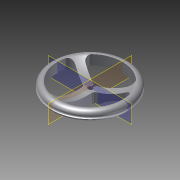
# Autodesk Inventor part: Rueda1
Saved by Autodesk Inventor 2012 (Build 160160000, 160)
## iProperties
Created: 2012-12-03
Part Number: Rueda1
Material: Default
Document SubType Name: Modeling
Designer: ALUMNO
Density: 1 g/cm^3
Author: ALUMNO
Autodesk Inventor part; units mm, degrees
ref_plane "XY Plane" through (0, 0, 0) normal (0, 0, 1) x (1, 0, 0)
sketch "Sketch1" plane through (0, 0, 0) normal (0, 0, 1) x (1, 0, 0)
  line L0 (-20, 0) -> (20, 0) construction
  line L1 (-1.118, -1) -> (1.118, -1)
  line L2 (0, -3.5) -> (0, -10.5) construction
  line L3 (0, 42) -> (0, -42) construction
  line L4 (3, -1.8028) -> (3, -19.7737)
  line L5 (-3, -1.8028) -> (-3, -19.7737)
  line L6 (3.0311, 1.75) -> (9.0933, 5.25) construction
  line L7 (-3.0311, 1.75) -> (-9.0933, 5.25) construction
  line L8 (3.4347, -0.6728) -> (18.3556, 7.9418)
  line L9 (1.1347, 3.3109) -> (16.0556, 11.9255)
  arc A0 (3, -19.7737) -> (18.3556, 7.9418) centre (0, 0) ccw
  line L10 (-16.0556, 11.9255) -> (-1.1347, 3.3109)
  line L11 (-18.3556, 7.9418) -> (-3.4347, -0.6728)
  arc A1 (16.0556, 11.9255) -> (-16.0556, 11.9255) centre (0, 0) ccw
  arc A2 (-18.3556, 7.9418) -> (-3, -19.7737) centre (0, 0) ccw
  arc A3 (-3.4347, -0.6728) -> (-3, -1.8028) centre (0, 0) ccw
  arc A4 (3, -1.8028) -> (3.4347, -0.6728) centre (0, 0) ccw
  line L12 (0, 0) -> (2.0417, 7.6198) construction
  line L13 (0, 0) -> (-1.8775, 7.0067) construction
  line L14 (0.3882, 1.4489) -> (0.9059, 3.3807)
  line L15 (-0.3882, 1.4489) -> (-0.9059, 3.3807)
  arc A5 (1.1347, 3.3109) -> (0.9059, 3.3807) centre (0, 0) ccw
  arc A6 (-0.9059, 3.3807) -> (-1.1347, 3.3109) centre (0, 0) ccw
  arc A7 (1.118, -1) -> (0.3882, 1.4489) centre (0, 0) ccw
  arc A8 (-0.3882, 1.4489) -> (-1.118, -1) centre (0, 0) ccw
  circle A9 centre (0, 0) radius 30
  dimension "d3" = 1
  dimension "d4" = 3
  dimension "d5" = 3
  dimension "d8" = 360
  dimension "d10" = 2.3
  dimension "d11" = 2.3
  dimension "d12" = 2.3
  dimension "d13" = 2.3
  dimension "d14" = 20
  dimension "d15" = 20
  dimension "d16" = 20
  dimension "d17" = 3.5
  dimension "d18" = 3.5
  dimension "d19" = 15
  dimension "d20" = 15
  dimension "d21" = 3.5
  dimension "d22" = 3.5
  dimension "d23" = 1.5
  dimension "d24" = 1.5
  dimension "d25" = 60
  constraints: 30 end point, 21 point on circle, 10 centre point, 7 parallel, 5 point on line, 4 coincident, 1 collinear, 1 horizontal, 1 midpoint, 1 perpendicular, 10 other
  measures "d3" distance between parallel lines of L1 L0
  measures "d4" distance between parallel lines of L4 L2
  measures "d5" distance between parallel lines of L2 L5
  measures "d10" distance between parallel lines of L9 L6
  measures "d11" distance between parallel lines of L8 L6
  measures "d12" distance between parallel lines of L10 L7
  measures "d13" distance between parallel lines of L7 L11
  measures "d14" radius of A1
  measures "d15" radius of A0
  measures "d16" radius of A2
  measures "d17" radius of A4
  measures "d18" radius of A3
  measures "d19" angle of L3 L12
  measures "d20" angle of L3 L13
  measures "d21" radius of A5
  measures "d22" radius of A6
  measures "d23" radius of A8
  measures "d24" radius of A7
  measures "d25" diameter of A9
extrude "Extrusion1" add sketch "Sketch1" along normal blind 15
sketch "Sketch2" plane through (0, 0, 0) normal (1, 0, 0) x (0, 1, 0)
  line L0 (0, 59.2166) -> (0, -51.2187) construction
  line L1 (1.4489, 0) -> (-1, 0) construction
  line L2 (0, 0) -> (3.3512, 0)
  line L3 (3.5, 5.9982) -> (0, 5.9982)
  line L4 (0, 5.9982) -> (0, 0)
  line L5 (3.5, 4.1688) -> (3.5, 5.9982)
  arc A0 (3.3512, 0) -> (3.5, -0.0058) centre (5.1259, 43.4402) ccw
  arc A1 (3.3512, 0) -> (7.526, 1.4627) centre (4.1095, 4.525) ccw
  arc A2 (3.5, 5.9982) -> (19.2603, 9.7212) centre (5.9262, 30.9473) ccw
  arc A3 (20.602, 4.0379) -> (7.526, 1.4627) centre (21.5858, -35.4422) ccw
  arc A4 (23.4353, 8.024) -> (23.4353, 6.0519) centre (23.602, 7.0379) ccw
  arc A5 (20.602, 4.0379) -> (23.4353, 6.0519) centre (20.602, 7.0379) ccw
  arc A6 (23.4353, 8.024) -> (18.8167, 9.4489) centre (20.602, 7.0379) ccw
  point P0 (3.5, 2.6464)
  point P1 (3.3512, -0.5504)
  dimension "d33" = 3.5
  dimension "d62" = 2
  constraints: 16 point on circle, 8 end point, 7 centre point, 2 parallel, 2 point on line, 1 horizontal, 1 perpendicular
  measures "d33" distance of L3.start L3.end
  measures "d62" diameter of A4
revolve "Revolution1" cut sketch "Sketch2" angle 360 about axis through (0, 0, 0) along (0, 0, -1) keep common part contours L4 L3 A2 A6 A4 A5 A3 A1 L2
fillet "Fillet10" radius 1 6 edges at (3.4347, -0.6728, 2.9991) (3, -1.8028, 2.9991) (-3.4347, -0.6728, 2.9991) (-3, -1.8028, 2.9991) (-1.1347, 3.3109, 2.9991) (1.1347, 3.3109, 2.9991)
fillet "Fillet11" radius 3 6 edges at (-18.3556, 7.9418, 6.9976) (-16.0556, 11.9255, 6.9976) (16.0556, 11.9255, 6.9976) (18.3556, 7.9418, 6.9976) (3, -19.7737, 6.9976) (-3, -19.7737, 6.9976)
equation "\"d5\" = d4"
equation "\"d11\" = d10"
equation "\"d12\" = d10"
equation "\"d13\" = d10"
equation "\"d15\" = d14"
equation "\"d18\" = d17"
equation "\"d20\" = d19"
equation "\"d21\" = d17"
equation "\"d22\" = d17"
equation "\"d24\" = d23"
body "Solid1"
